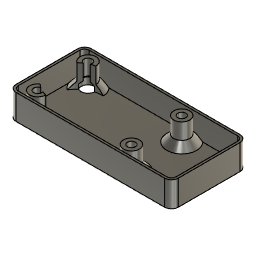
EDiceBottom (Autodesk Fusion 360 design; units mm, degrees)
Autodesk Fusion 360 part; units mm, degrees
sketch "Skizze1" plane through (0, 0, 0) normal (0, 0, 1) x (1, 0, 0)
  line L0 (0, 0) -> (71, 0)
  line L1 (71, 0) -> (71, 16.5)
  line L2 (71, 16.5) -> (0, 16.5)
  line L3 (0, 16.5) -> (0, 0)
  dimension "d1" = 71
  dimension "d2" = 16.5
  constraint horizontal L0
  constraint vertical L1
  constraint horizontal L2
  constraint vertical L3
  constraint coincident L0.start L3.end
  measures "d1" distance of L0.start L0.end
  measures "d2" distance of L0.end L1.end
extrude "Extrusion1" add sketch "Skizze1" along normal blind 1
sketch "Skizze2" plane through (0, 0, 1) normal (0, 0, 1) x (-1, 0, 0)
  line L0 (0, -16.5) -> (0, 0)
  line L1 (0, 0) -> (-71, 0)
  line L2 (-71, 0) -> (-71, -16.5)
  line L3 (-71, -16.5) -> (0, -16.5)
  line L4 (0, 0) -> (0, -16.5)
  line L5 (-71, -16.5) -> (0, -16.5)
  line L6 (-71, -16.5) -> (-71, 0)
  line L7 (-71, 0) -> (-70, 0)
  line L8 (-70, -15.5) -> (-70, 0)
  line L9 (-70, -15.5) -> (-1, -15.5)
  line L10 (-1, -15.5) -> (-1, 0)
  line L11 (-1, 0) -> (0, 0)
  dimension "d5" = 1
  dimension "d6" = 1
  dimension "d7" = 1
  constraint coincident L0.end L1.start
  constraint coincident L0.start L3.end
  constraint coincident L2.end L3.start
  constraint coincident L1.end L2.start
  constraint coincident L1 L7.end
  constraint perpendicular L6 L7
  constraint perpendicular L7 L8
  constraint perpendicular L8 L9
  constraint coincident L1 L10.end
  constraint perpendicular L1 L10
  measures "d5" distance of L10.end L0.end
  measures "d6" distance of L1.end L7.end
  measures "d7" distance of L2.end L9
extrude "Extrusion2" add sketch "Skizze2" along normal blind 10 contours L0 L1 L2 L3 L4 L5 L6 L7 L8 L9 L10 L11
sketch "Skizze3" plane through (0, 0, 1) normal (0, 0, 1) x (-1, 0, 0)
  line L0 (-1, -15.5) -> (-1, 0)
  line L1 (-1, 0) -> (-70, 0)
  line L2 (-70, 0) -> (-70, -15.5)
  line L3 (-70, -15.5) -> (-1, -15.5)
  circle A0 centre (-7, -11) radius 3.5
  circle A1 centre (-48, -11) radius 3.5
  dimension "d10" = 7
  dimension "d11" = 7
  dimension "d12" = 11
  dimension "d13" = 11
  dimension "d14" = 41
  dimension "d15" = 7
  measures "d10" diameter of A0
  measures "d11" diameter of A1
  measures "d12" distance of L1 A0.centre
  measures "d13" distance of L1 A1.centre
  measures "d14" distance of A0.centre A1.centre
  measures "d15" horizontal distance of origin A0.centre
extrude "Extrusion3" add sketch "Skizze3" along normal blind 10 contours A0 | A1
sketch "Skizze4" plane through (0, 0, 11) normal (0, 0, 1) x (-1, 0, 0)
  circle A0 centre (-7, -11) radius 3.5
  circle A1 centre (-48, -11) radius 3.5
  point P0 (-7, -11)
  point P1 (-48, -11)
  constraint coincident P0 A0.centre
  constraint coincident P1 A1.centre
hole "Bohrung1" at (7, 11, 11) at (48, 11, 11) direction (0, 0, -1) diameter 3.5 end through all
sketch "Skizze5" plane through (0, 0, 11) normal (0, 0, 1) x (-1, 0, 0)
  circle A0 centre (-7, -11) radius 1.75
  circle A1 centre (-7, -11) radius 3.5
  circle A2 centre (-13, 0) radius 11.25
  line L0 (-1, 0) -> (-70, 0)
  dimension "d21" = 22.5
  dimension "d22" = 13
  constraint coincident A2.centre L0
  measures "d21" diameter of A2
  measures "d22" distance of origin A2.centre
extrude "Extrusion4" cut sketch "Skizze5" against normal blind 10 contours A0 A1 A2 picked at (-9.2351, -9.948)
fillet "Abrundung1" radius 2 2 edges at (1, 15.5, 6) (70, 15.5, 6)
fillet "Abrundung2" radius 3 2 edges at (71, 16.5, 5.5) (0, 16.5, 5.5)
sketch "Skizze7" plane through (0, 0, 0) normal (0, 0, -1) x (1, 0, 0)
  arc A0 (0, -13.5) -> (3, -16.5) centre (3, -13.5) ccw
  line L0 (3, -16.5) -> (68, -16.5)
  arc A1 (68, -16.5) -> (71, -13.5) centre (68, -13.5) ccw
  line L1 (71, -13.5) -> (71, 0)
  line L2 (71, 0) -> (0, 0)
  line L3 (0, 0) -> (0, -13.5)
  circle A2 centre (7, -11) radius 1.75
  circle A3 centre (48, -11) radius 1.75
  circle A4 centre (7, -11) radius 1.75
  circle A5 centre (48, -11) radius 1.75
  point P0 (7, -11)
  point P1 (48, -11)
  constraint coincident P0 A2.centre
  constraint coincident P1 A3.centre
hole "Bohrung3" at (7, 11, 0) at (48, 11, 0) direction (0, 0, 1) diameter 6 depth 3 tip angle 180
chamfer "Fase1" distance 3 angle 45 2 edges at (5.324, 14.0726, 1) (51.2631, 9.7343, 1)
chamfer "Fase3" distance 1.25 angle 45 2 edges at (6.162, 12.5363, 3) (46.3684, 11.6328, 3)
mirror "Spiegeln1" about plane through (0, 0, 0) normal (0, 1, 0) of bodies 1 merged
equation "d1 = 65 mm + 2 mm + 4 mm"
equation "d2 = 15 mm + 1.5 mm"
